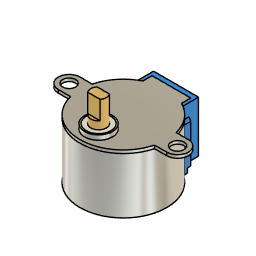
Airspeed Indicator v2 (Autodesk Fusion 360 archive; units mm, degrees)
design "28BYJ-48_5VDC"
Autodesk Fusion 360 part; units mm, degrees
note: some values were not read from the file. Set by a fixed rule: which face or edge a step refers to.
sketch "Sketch1" plane through (0, 0, 0) normal (0, 0, 1) x (1, 0, 0)
  circle A0 centre (0, 0) radius 14 construction
  line L0 (7.25, 11.9765) -> (-7.25, 11.9765) construction
  line L1 (-7.25, 11.9765) -> (-7.25, 17)
  line L2 (-7.25, 17) -> (7.25, 17)
  line L3 (7.25, 17) -> (7.25, 11.9765)
  line L4 (7.25, 11.9765) -> (-7.25, 17) construction
  line L5 (-7.25, 11.9765) -> (7.25, 17) construction
  arc A1 (-7.25, 11.9765) -> (7.25, 11.9765) centre (0, 0) ccw
  point P0 (0, 14.4883)
  dimension "d1" = 28
  dimension "d4" = 31
  dimension "d5" = 14.5
  constraint coincident A0.centre A1.centre
  constraint horizontal L0
  constraint perpendicular L0 L1
  constraint parallel L0 L2
  constraint parallel L1 L3
  constraint coincident L4 P0
  constraint coincident L5 P0
  constraint vertical A0.centre P0
  constraint coincident A0 L0.start
  measures "d1" diameter of A0
  measures "d5" distance of L1.end L2.end
extrude "Extrude1" add sketch "Sketch1" along normal blind 19 makes body 1
sketch "Sketch2" plane through (0, 0, 0) normal (0, 0, -1) x (1, 0, 0)
  line L0 (-7.25, -11.9765) -> (-7.25, -17)
  line L1 (-7.25, -17) -> (7.25, -17)
  line L2 (7.25, -17) -> (7.25, -11.9765)
  arc A0 (7.25, -11.9765) -> (-7.25, -11.9765) centre (0, 0) ccw
  line L3 (-8.75, -10.9287) -> (8.75, -10.9287) construction
  line L4 (8.75, -10.9287) -> (8.75, -14) construction
  line L5 (8.75, -14) -> (-8.75, -14) construction
  line L6 (-8.75, -14) -> (-8.75, -10.9287)
  line L7 (-8.75, -10.9287) -> (8.75, -14) construction
  line L8 (8.75, -10.9287) -> (-8.75, -14) construction
  line L9 (8.75, -13) -> (-8.75, -13) construction
  line L10 (-8.75, -13) -> (-7.25, -14)
  line L11 (8.75, -13) -> (7.25, -14)
  line L12 (8.75, -13) -> (8.75, -10.9287)
  line L13 (-8.75, -13) -> (-8.75, -10.9287)
  line L14 (-7.25, -14) -> (-7.25, -11.9765)
  line L15 (7.25, -14) -> (7.25, -11.9765)
  arc A1 (7.25, -11.9765) -> (8.75, -10.9287) centre (0, 0) ccw
  arc A2 (-8.75, -10.9287) -> (-7.25, -11.9765) centre (0, 0) ccw
  point P0 (0, -12.4644)
  dimension "d8" = 17.5
  dimension "d9" = 3
  dimension "d10" = 4
  constraint horizontal L3
  constraint perpendicular L3 L4
  constraint parallel L3 L5
  constraint parallel L4 L6
  constraint coincident L7 P0
  constraint coincident L8 P0
  constraint vertical A0.centre P0
  constraint coincident L4 L9.start
  constraint coincident L6 L9.end
  constraint perpendicular L6 L9
  constraint coincident L5 L10.end
  constraint coincident L0 L10.end
  constraint coincident L5 L11.end
  constraint coincident L2 L11.end
  constraint coincident A0 L3.end
  constraint coincident L0.start A0.end
  constraint coincident L2.end A0.start
  constraint concentric A0 A1
  constraint concentric A0 A2
  measures "d8" distance of L4.end L5.end
  measures "d9" distance of L1 L5
  measures "d10" distance of L1 L9
extrude "Extrude2" add sketch "Sketch2" against normal blind 15 contours L0 A0 L6 L10 L13 L14 A2 | L2 A0 L11 L12 L15 A1 bodies 1
sketch "Sketch3" plane through (0, 0, 0) normal (0, 0, -1) x (1, 0, 0)
  line L0 (-7.25, -14) -> (-7.25, -17)
  line L1 (-7.25, -17) -> (7.25, -17)
  line L2 (7.25, -17) -> (7.25, -14)
  line L3 (7.25, -14) -> (8.75, -13)
  line L4 (8.75, -13) -> (8.75, -10.9287)
  arc A0 (8.75, -10.9287) -> (-8.75, -10.9287) centre (0, 0) ccw
  line L5 (-8.75, -10.9287) -> (-8.75, -13)
  line L6 (-8.75, -13) -> (-7.25, -14)
  line L7 (8.75, -11.9287) -> (8.75, -13)
  line L8 (8.75, -13) -> (7.25, -14)
  line L9 (7.25, -14) -> (7.25, -17)
  line L10 (7.25, -17) -> (-7.25, -17)
  line L11 (-7.25, -17) -> (-7.25, -14)
  line L12 (-7.25, -14) -> (-8.75, -13)
  line L13 (-8.75, -13) -> (-8.75, -11.9287)
  arc A1 (-8.75, -10.9287) -> (8.75, -10.9287) centre (0, 0) ccw
  arc A2 (-8.75, -11.9287) -> (8.75, -11.9287) centre (0, 0) ccw
  line L14 (-1.5, -12.5) -> (1.5, -12.5) construction
  line L15 (1.5, -12.5) -> (1.5, -15.5) construction
  line L16 (1.5, -15.5) -> (-1.5, -15.5)
  line L17 (-1.5, -15.5) -> (-1.5, -12.5) construction
  line L18 (-1.5, -12.5) -> (1.5, -15.5) construction
  line L19 (1.5, -12.5) -> (-1.5, -15.5) construction
  line L20 (1.5, -15.5) -> (1.5, -13.9194)
  line L21 (-1.5, -15.5) -> (-1.5, -13.9194)
  point P0 (0, -14)
  dimension "d13" = 1
  dimension "d14" = 1
  dimension "d15" = 3
  constraint coincident L4 L7.start
  constraint coincident L3.end L4.start
  constraint parallel L4 L7
  constraint coincident L2.end L3.start
  constraint coincident L1.end L2.start
  constraint coincident L0.end L1.start
  constraint coincident L0.start L6.end
  constraint coincident L5.end L6.start
  constraint coincident L5 L13.end
  constraint parallel L5 L13
  constraint coincident L4.end A0.start
  constraint coincident A0.centre A1.centre
  constraint coincident A0.end L5.start
  constraint horizontal L14
  constraint perpendicular L14 L15
  constraint parallel L14 L16
  constraint parallel L15 L17
  constraint coincident L18 P0
  constraint coincident L19 P0
  constraint vertical A0.centre P0
  constraint midpoint A1 P0
  constraint equal L15 L16
  constraint coincident A1 L20.end
  constraint coincident L15 L20.end
  constraint coincident A1 L21.end
  constraint coincident L17 L21.end
  measures "d13" distance of L7.start L4.end
  measures "d14" distance of L13.end A0.end
  measures "d15" distance of L15.end L16.end
extrude "Extrude3" cut sketch "Sketch3" against normal blind 2.5 contours L0 L1 L2 L3 L4 L5 L6 L7 L8 L9 L10 L11 L12 L13 A2 L16 L20 L21 | A1 A2 L20 L21 | A2 L16 L20 L21 bodies 1
extrude "Extrude4" cut sketch "Sketch3" against normal blind 1 contours L5 A1 A2 L21 | A1 A2 L20 L21 | L4 A1 A2 L20 bodies 1
sketch "Sketch4" plane through (0, 17, 0) normal (0, 1, 0) x (-1, 0, 0)
  line L0 (-7.25, 2.5) -> (7.25, 2.5)
  line L1 (7.25, 2.5) -> (7.25, 19)
  line L2 (7.25, 19) -> (-7.25, 19)
  line L3 (-7.25, 19) -> (-7.25, 2.5)
  line L4 (0, 19) -> (0, 2.5) construction
  line L5 (-3, 16) -> (3, 16)
  arc A0 (3, 16) -> (3, 17) centre (3, 16.5) ccw
  line L6 (3, 17) -> (-3, 17)
  arc A1 (-3, 17) -> (-3, 16) centre (-3, 16.5) ccw
  line L7 (-3, 16.5) -> (3, 16.5) construction
  point P0 (0, 16.5)
  dimension "d21" = 1
  dimension "d22" = 7
  dimension "d23" = 2
  constraint midpoint L2 L4.start
  constraint midpoint L0 L4.end
  constraint tangent L5 A0
  constraint tangent A0 L6
  constraint parallel L5 L6
  constraint tangent L6 A1
  constraint tangent L5 A1
  constraint perpendicular L4 L7
  constraint coincident L4 P0
  constraint midpoint L7 P0
  measures "d21" distance of L5 L6
  measures "d23" distance of L2 L6
extrude "Extrude5" cut sketch "Sketch4" against normal blind 0.5 contours L5 A0 L6 A1 bodies 1
sketch "Sketch5" plane through (0, 16.5, 0) normal (0, 1, 0) x (-1, 0, 0)
  arc A0 (-3, 17) -> (-3, 16) centre (-3, 16.5) ccw
  line L0 (-3, 16) -> (3, 16)
  arc A1 (3, 16) -> (3, 17) centre (3, 16.5) ccw
  line L1 (3, 17) -> (-3, 17)
  line L2 (-3.5, 16.5) -> (3.5, 16.5) construction
  line L3 (0, 17) -> (0, 16) construction
  circle A2 centre (0, 16.5) radius 0.5
  circle A3 centre (-2.4, 16.5) radius 0.5
  circle A4 centre (-1.2, 16.5) radius 0.5
  circle A5 centre (1.2, 16.5) radius 0.5
  circle A6 centre (2.4, 16.5) radius 0.5
  dimension "d26" = 1
  dimension "d27" = 1.2
  dimension "d28" = 1.2
  dimension "d29" = 1.2
  dimension "d30" = 1.2
  constraint midpoint A0 L2.start
  constraint midpoint A1 L2.end
  constraint midpoint L1 L3.start
  constraint midpoint L0 L3.end
  constraint coincident L2 A2.centre
  constraint coincident L3 A2.centre
  constraint coincident L2 A3.centre
  constraint coincident L2 A4.centre
  constraint coincident L2 A5.centre
  constraint coincident L2 A6.centre
  constraint equal A2 A3
  constraint equal A2 A4
  constraint equal A2 A5
  constraint equal A2 A6
  measures "d26" diameter of A2
  measures "d27" distance of A2.centre A4.centre
  measures "d28" distance of A3.centre A4.centre
  measures "d29" distance of A2.centre A5.centre
  measures "d30" distance of A5.centre A6.centre
extrude "Extrude6" add sketch "Sketch5" along normal blind 0.5 separate body contours A3 | A4 | A2 | A5 | A6 makes body 2 at (-0.4845, 16.8333, 16.6234) makes body 3 at (-0.7393, 16.8333, 16.6942) makes body 4 at (0.7155, 16.8333, 16.6234) makes body 5 at (-1.9393, 16.8333, 16.6942) makes body 6 at (2.8607, 16.8333, 16.6942)
sketch "Sketch6" plane through (0, 0, 19) normal (0, 0, 1) x (-1, 0, 0)
  line L0 (7.25, -17) -> (7.25, -11.9765)
  arc A0 (7.25, -11.9765) -> (-7.25, -11.9765) centre (0, 0) ccw
  line L1 (-7.25, -11.9765) -> (-7.25, -17)
  line L2 (-7.25, -17) -> (7.25, -17)
  line L3 (6.25, -12.5275) -> (6.25, -15.5)
  line L4 (6.25, -15.5) -> (-6.2374, -15.5)
  line L5 (-6.2374, -15.5) -> (-6.2374, -12.5337)
  circle A1 centre (0, 0) radius 14
  dimension "d33" = 1
  dimension "d34" = 1.0126
  dimension "d35" = 1.5
  constraint parallel L0 L3
  constraint perpendicular L3 L4
  constraint perpendicular L4 L5
  constraint concentric A0 A1
  constraint equal A0 A1
  constraint coincident L3.start A1
  constraint coincident L5.end A1
  measures "d33" distance of L0 L3
  measures "d34" distance of L1 L5
  measures "d35" distance of L2 L4
extrude "Extrude7" cut sketch "Sketch6" against normal blind 1 contours A0 A1 | L3 L4 L5 A1 bodies 1
sketch "Sketch7" plane through (0, 0, 18) normal (0, 0, 1) x (-1, 0, 0)
  arc A0 (-7.25, -11.9765) -> (-6.2374, -12.5337) centre (0, 0) ccw
  line L0 (-6.2374, -12.5337) -> (-6.2374, -15.5)
  line L1 (-6.2374, -15.5) -> (6.25, -15.5)
  line L2 (6.25, -15.5) -> (6.25, -12.5275)
  arc A1 (6.25, -12.5275) -> (7.25, -11.9765) centre (0, 0) ccw
  arc A2 (7.25, -11.9765) -> (-7.25, -11.9765) centre (0, 0) ccw
  line L3 (3, -17) -> (-3, -17) construction
  line L4 (0, -17) -> (0, 14) construction
  line L5 (14, 0) -> (-14, 0) construction
  circle A3 centre (17.5, 0) radius 2.1
  circle A4 centre (-17.5, 0) radius 2.1
  line L6 (21, -3.5) -> (13.5554, -3.5)
  line L7 (13.5554, -3.5) -> (13.5554, 3.5)
  line L8 (13.5554, 3.5) -> (21, 3.5)
  line L9 (21, 3.5) -> (21, -3.5)
  line L10 (-13.5554, 3.5) -> (-21, 3.5)
  line L11 (-21, 3.5) -> (-21, -3.5)
  line L12 (-21, -3.5) -> (-13.5554, -3.5)
  line L13 (-13.5554, -3.5) -> (-13.5554, 3.5)
  circle A5 centre (17.5, 0) radius 3.5
  circle A6 centre (-17.5, 0) radius 3.5
  dimension "d46" = 4.2
  dimension "d47" = 35
  dimension "d48" = 17.5
  dimension "d49" = 7
  dimension "d50" = 42
  constraint midpoint L3 L4.start
  constraint midpoint A2 L4.end
  constraint horizontal L5
  constraint coincident A0.centre L5
  constraint coincident A2 L5.start
  constraint coincident A2 L5.end
  constraint coincident L5 A3.centre
  constraint coincident L5 A4.centre
  constraint equal A3 A4
  constraint horizontal L6
  constraint vertical L7
  constraint horizontal L8
  constraint vertical L9
  constraint symmetric L5 L6 L8
  constraint horizontal L10
  constraint vertical L11
  constraint horizontal L12
  constraint vertical L13
  constraint symmetric L5 L10 L12
  constraint equal L7 L11
  constraint coincident A2 L6.end
  constraint coincident A2 L12.end
  constraint symmetric L4 L9 L11
  constraint tangent L8 A5
  constraint tangent L9 A5
  constraint tangent L6 A5
  constraint tangent L12 A6
  constraint tangent L11 A6
  constraint tangent L10 A6
  measures "d46" diameter of A3
  measures "d47" distance of A3.centre A4.centre
  measures "d48" distance of L4 A3.centre
  measures "d49" distance of L6.start L8.end
  measures "d50" distance of L9 L11
extrude "Extrude8" add sketch "Sketch7" along normal blind 1 separate body contours A0 L0 L1 L2 A1 A2 L7 L13 | A2 L12 A6 | A2 L13 | A2 L10 A6 | A6 | A2 L8 A5 | A2 L7 | A2 L6 A5 | A5 makes body 7
sketch "Sketch8" plane through (0, 0, 19) normal (0, 0, 1) x (-1, 0, 0)
  circle A0 centre (17.5, 0) radius 2.1
  circle A1 centre (-17.5, 0) radius 2.1
  arc A2 (13.5554, 3.5) -> (-13.5554, 3.5) centre (0, 0) ccw
  line L0 (-13.5554, 3.5) -> (-17.5, 3.5)
  arc A3 (-17.5, 3.5) -> (-17.5, -3.5) centre (-17.5, 0) ccw
  line L1 (-17.5, -3.5) -> (-13.5554, -3.5)
  arc A4 (-13.5554, -3.5) -> (-6.2374, -12.5337) centre (0, 0) ccw
  line L2 (-6.2374, -12.5337) -> (-6.2374, -15.5)
  line L3 (-6.2374, -15.5) -> (6.25, -15.5)
  line L4 (6.25, -15.5) -> (6.25, -12.5275)
  arc A5 (6.25, -12.5275) -> (13.5554, -3.5) centre (0, 0) ccw
  line L5 (13.5554, -3.5) -> (17.5, -3.5)
  arc A6 (17.5, -3.5) -> (17.5, 3.5) centre (17.5, 0) ccw
  line L6 (17.5, 3.5) -> (13.5554, 3.5)
  circle A7 centre (0, 8) radius 4.5
  circle A8 centre (0, 8) radius 4
  dimension "d53" = 9
  dimension "d54" = 8
  dimension "d55" = 8
  constraint vertical A2.centre A7.centre
  constraint concentric A7 A8
  measures "d53" diameter of A7
  measures "d54" distance of A2.centre A7.centre
  measures "d55" diameter of A8
extrude "Extrude9" add sketch "Sketch8" along normal blind 1.5 contours A7 bodies 7
extrude "Extrude10" add 1 faces at (0.3559, -8.9069, 19) along direction (0, 0, 1) blind 1.5 separate body on bodies 7 makes body 8
sketch "Sketch9" plane through (0, 0, 20.5) normal (0, 0, 1) x (-1, 0, 0)
  circle A0 centre (0, 8) radius 4
  circle A1 centre (0, 8) radius 2.5
  dimension "d60" = 5
  constraint concentric A0 A1
  measures "d60" diameter of A1
extrude "Extrude11" add sketch "Sketch9" along normal blind 2.5 contours A1 bodies 8
sketch "Sketch10" plane through (0, 0, 23) normal (0, 0, 1) x (-1, 0, 0)
  circle A0 centre (0, 8) radius 2.5
  line L0 (-2, 9.5) -> (2, 9.5)
  line L1 (2, 9.5) -> (2, 6.5)
  line L2 (2, 6.5) -> (-2, 6.5)
  line L3 (-2, 6.5) -> (-2, 9.5)
  line L4 (-2, 9.5) -> (2, 6.5) construction
  line L5 (2, 9.5) -> (-2, 6.5) construction
  point P0 (0, 8)
  dimension "d63" = 3
  constraint horizontal L0
  constraint perpendicular L0 L1
  constraint parallel L0 L2
  constraint parallel L1 L3
  constraint coincident A0 L0.start
  constraint coincident L4 P0
  constraint coincident L5 P0
  constraint coincident P0 A0.centre
  measures "d63" distance of L0.start L2.end
extrude "Extrude12" add sketch "Sketch10" along normal blind 6 contours A0 L1 | L0 L1 L2 L3 | A0 L3 bodies 8
sketch "Sketch11" plane through (0, 0, 0) normal (0, 0, -1) x (1, 0, 0)
  circle A0 centre (0, 0) radius 14
  line L0 (-14, -14) -> (14, -14) construction
  line L1 (14, -14) -> (14, 14) construction
  line L2 (14, 14) -> (-14, 14) construction
  line L3 (-14, 14) -> (-14, -14) construction
  dimension "d66" = 2
  text T0 "STEP MOTOR\n\n\n28BYJ-48" font "Arial" height 2 align centre middle in box 28 x 28 at (-14, -14) x (1, 0) y (0, 1) spacing 1 kerned
  constraint tangent A0 L2
  constraint tangent A0 L3
  constraint tangent A0 L1
  constraint tangent A0 L0
  constraint vertical L1
extrude "Extrude13" cut sketch "Sketch11" against normal blind 0.5 text T0 bodies 1
extrude "Extrude14" add 17 faces at (-8.1447, -4.6404, 0.5) (-6.5543, -4.8581, 0.5) (-5.3511, -4.6544, 0.5) (-3.493, -4.6985, 0.5) (0.8236, -4.9068, 0.5) (1.356, -4.7949, 0.5) (4.1942, -4.2701, 0.5) (5.1855, -4.7949, 0.5) (7.4307, -4.6448, 0.5) (4.0491, 4.2456, 0.5) (5.4838, 4.6007, 0.5) (2.392, 4.9172, 0.5) (1.6585, 4.5957, 0.5) (-0.7049, 4.2674, 0.5) (-2.7794, 4.7076, 0.5) (-3.6785, 4.6007, 0.5) (-5.5412, 5.6035, 0.5) along direction (0, 0, -1) blind 0.5 separate body on bodies 1 makes body 9 at (-3.6785, 4.6007, 0.5) makes body 10 at (-0.7049, 4.2674, 0.5) makes body 11 at (2.392, 4.8349, 0.3333) makes body 12 at (4.0491, 4.2456, 0.5) makes body 13 at (5.1855, -4.7949, 0.5) makes body 14 at (1.356, -4.7949, 0.5) makes body 15 at (-3.493, -4.6985, 0.5) makes body 16 at (-6.6426, -4.2701, 0.3333) makes body 17 at (-8.1447, -4.6404, 0.5) makes body 18 at (-5.3511, -4.6544, 0.5) makes body 19 at (0.8236, -4.9068, 0.5) makes body 20 at (4.0177, -4.2701, 0.3333) makes body 21 at (7.4307, -4.6448, 0.5) makes body 22 at (5.4838, 4.6007, 0.5) makes body 23 at (1.6585, 4.5957, 0.5) makes body 24 at (-2.7794, 4.7076, 0.5) makes body 25 at (-5.5412, 5.6035, 0.5)
equation "d28 = d27"
equation "d29 = d27"
equation "d30 = d27"
equation "d48 = d47 / 2"
